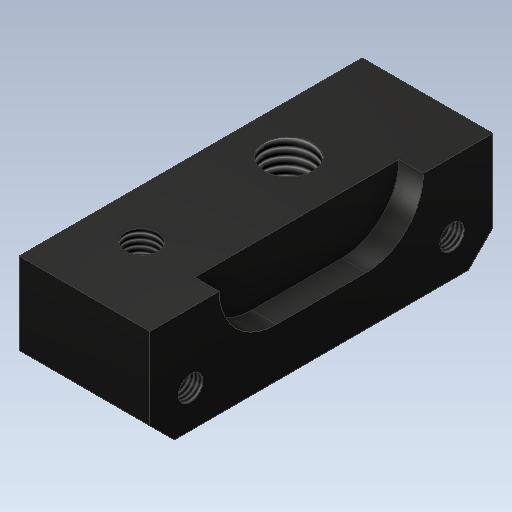
# Autodesk Inventor part: 33_ekstruder1
Saved by Autodesk Inventor 2020.2 (Build 242310000, 310)
## iProperties
Created: 2017-11-11
Part Number: 33_ekstruder1
Material: Ogólny
Document SubType Name: Modeling
Designer: Haras
Density: 1 g/cm^3
Appearance: Domyślna
Author: Haras
Autodesk Inventor part; units mm, degrees
ref_plane "YZ Plane" through (0, 0, 0) normal (1, 0, 0) x (0, 1, 0)
ref_plane "XZ Plane" through (0, 0, 0) normal (0, 1, 0) x (-1, 0, 0)
ref_plane "XY Plane" through (0, 0, 0) normal (0, 0, 1) x (1, 0, 0)
sketch "Szkic1" plane through (0, 0, 0) normal (1, 0, 0) x (0, 1, 0)
  line L0 (13, 21) -> (0, 21)
  line L1 (0, 21) -> (0, -21)
  line L2 (0, -21) -> (13, -21)
  line L3 (13, -21) -> (13, 21)
  line L4 (0, 0) -> (13, 0) construction
  dimension "d0" = 42
  dimension "d1" = 13
  constraints: 10 end point, 2 horizontal, 2 midpoint, 2 parallel, 1 perpendicular
  measures "d0" distance of L0.end L1.end
  measures "d1" distance of L1.end L2.end
extrude "Wyciągnięcie proste3" add sketch "Szkic1" along normal blind 16
sketch "Szkic4" plane through (16, 0, 0) normal (1, 0, 0) x (0, 0, -1)
  line L0 (-12.5, 13) -> (12.5, 13)
  line L1 (12.5, 13) -> (12.5, 6)
  line L2 (12.5, 6) -> (-12.5, 6)
  line L3 (-12.5, 6) -> (-12.5, 13)
  line L4 (0, 6) -> (0, 0) construction
  line L5 (21, 13) -> (-21, 13) projected
  point P0 (0, 13)
  dimension "d10" = 25
  dimension "d11" = 7
  constraints: 10 end point, 3 midpoint, 2 parallel, 1 horizontal, 1 perpendicular, 1 vertical
  measures "d10" distance of L1.end L2.end
  measures "d11" distance of L0.end L1.end
extrude "Wyciągnięcie proste4" cut sketch "Szkic4" against normal blind 3
fillet "Zaokrąglenie1" radius 7 2 edges at (14.5, 6, 12.5) (14.5, 6, -12.5)
sketch "Szkic5" plane through (16, 0, 0) normal (1, 0, 0) x (0, 0, -1)
  line L0 (0, 0) -> (0, 13) construction
  line L1 (-12.5, 13) -> (12.5, 13) projected
  line L2 (-21, 13) -> (-21, 0) projected
  line L3 (-21, 0) -> (21, 0) projected
  point P0 (-16, 4.5)
  point P1 (16, 4.5)
  dimension "d15" = 32
  dimension "d17" = 4.5
  constraints: 2 end point, 1 horizontal alignment, 1 midpoint, 1 symmetric about line
  measures "d15" distance of point (16, 4.5) point (-16, 4.5)
  measures "d17" distance from line of L3 point (-16, 4.5)
hole "Otwór1" at (16, 4.5, 16) at (16, 4.5, -16) direction (-1, 0, 0) diameter 3 end through all
chamfer "Faza1" distance 3 angle 45 2 edges at (8, 0, 21) (8, 0, -21)
sketch "Szkic6" plane through (0, 0, -18) normal (0, -1, 0) x (1, 0, 0)
  line L0 (0, -3) -> (16, -3) projected
  line L1 (0, 36) -> (0, 0) projected
  point P0 (0, 18)
  point P1 (6, 12)
  dimension "d28" = 15
  dimension "d29" = 6
  measures "d28" distance from line of L0 point (6, 12)
  measures "d29" distance from line of L1 point (6, 12)
hole "Otwór2" at (6, 0, -6) direction (0, 1, 0) diameter 6 end through all
sketch "Szkic7" plane through (0, 0, -18) normal (0, -1, 0) x (1, 0, 0)
  line L0 (16, 39) -> (0, 39) projected
  circle A0 centre (6, 12) radius 3 projected
  point P0 (0, 18)
  point P1 (6, 30)
  dimension "d37" = 9
  constraints: 1 vertical alignment
  measures "d37" distance from line of L0 point (6, 30)
hole "Otwór3" at (6, 0, 12) direction (0, 1, 0) diameter 4 end through all
thread "Gwint1" size "M6x1" class "6H" standard "ANSI Metric M Profile" full length
thread "Gwint2" size "M4x0.7" class "6H" standard "ANSI Metric M Profile" full length
thread "Gwint3" size "M3x0.5" class "6H" standard "ANSI Metric M Profile" full length
thread "Gwint4" size "M3x0.5" class "6H" standard "ANSI Metric M Profile" full length
